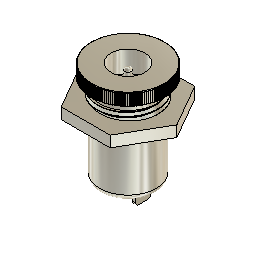
PowerConnector v3 (Autodesk Fusion 360 design; units mm, degrees)
Autodesk Fusion 360 part; units mm, degrees
sketch "Sketch1" plane through (0, 0, 0) normal (0, 0, 1) x (1, 0, 0)
  circle A0 centre (0, 0) radius 6
  circle A1 centre (0, 0) radius 2.75
  circle A2 centre (0, 0) radius 4.625
  dimension "d1" = 12
  dimension "d2" = 5.5
  dimension "d3" = 9.25
  constraint coincident A0.centre A1.centre
  constraint concentric A0 A1
  measures "d1" diameter of A0
  measures "d2" diameter of A1
  measures "d3" diameter of A2
extrude "Extrude1" add sketch "Sketch1" along normal blind 2 contours A0 | A1 | A2
extrude "Extrude2" add sketch "Sketch1" against normal blind 14.5 contours A1 | A2
fillet "Fillet1" radius 1 1 edges at (-4.312, 1.6725, -14.5)
sketch "Sketch2" plane through (0, 0, 2) normal (0, 0, 1) x (-1, 0, 0)
  circle A0 centre (0, 0) radius 6
  circle A1 centre (0, 0) radius 2.75
extrude "Extrude3" cut sketch "Sketch2" against normal blind 5 contours A1
ref_plane "WorkPlane1" through (0, 0, -3) normal (0, 0, 1) x (-1, 0, 0)
sketch "Sketch3" plane through (0, 0, -3) normal (0, 0, 1) x (1, 0, 0)
  circle A0 centre (0, 0) radius 0.5
  dimension "d15" = 1
  constraint coincident A0.centre origin
  measures "d15" diameter of A0
extrude "Extrude4" add sketch "Sketch3" along normal blind 4.5
fillet "Fillet2" radius 0.5 1 edges at (-0.4662, -0.1808, 1.5)
sketch "Sketch4" plane through (0, 0, -14.5) normal (0, 0, -1) x (1, 0, 0)
  circle A0 centre (0, 0) radius 3.625
  line L0 (-2.5, 1.25) -> (2.5, 1.25) construction
  line L1 (2.5, 1.25) -> (2.5, -1.25) construction
  line L2 (2.5, -1.25) -> (-2.5, -1.25) construction
  line L3 (-2.5, -1.25) -> (-2.5, 1.25) construction
  line L4 (-2.5, 1.25) -> (2.5, -1.25) construction
  line L5 (-2.5, 1.25) -> (-2, 1.25)
  line L6 (-2, 1.25) -> (-2, -1.25)
  line L7 (-2, -1.25) -> (-2.5, -1.25)
  line L8 (-2.5, -1.25) -> (-2.5, 1.25)
  line L9 (2.5, 1.25) -> (2, 1.25)
  line L10 (2, 1.25) -> (2, -1.25)
  line L11 (2, -1.25) -> (2.5, -1.25)
  line L12 (2.5, -1.25) -> (2.5, 1.25)
  dimension "d20" = 2.5
  dimension "d21" = 5
  dimension "d22" = 0.5
  dimension "d23" = 0.5
  constraint horizontal L0
  constraint vertical L1
  constraint horizontal L2
  constraint vertical L3
  constraint midpoint L4 A0.centre
  constraint coincident A0.centre origin
  constraint horizontal L5
  constraint vertical L6
  constraint horizontal L7
  constraint vertical L8
  constraint collinear L2 L7
  constraint horizontal L9
  constraint vertical L10
  constraint horizontal L11
  constraint vertical L12
  constraint coincident L2 L10.end
  measures "d20" distance of L0.start L2.end
  measures "d21" distance of L0.start L0.end
  measures "d22" distance of L0.start L5.end
  measures "d23" distance of L0.end L9.end
extrude "Extrude5" add sketch "Sketch4" along normal blind 2 contours L5 L6 L7 L8 | L9 L10 L11 L12
fillet "Fillet3" radius 0.5 4 edges at (-2.25, -1.25, -16.5) (-2.25, 1.25, -16.5) (2.25, -1.25, -16.5) (2.25, 1.25, -16.5)
sketch "Sketch5" plane through (0, 0, 2) normal (0, 0, 1) x (-1, 0, 0)
  circle A0 centre (0, 0) radius 2.75
  circle A1 centre (0, 0) radius 6
  circle A2 centre (0, 0) radius 6
  line L0 (0, 0) -> (-6, 0) construction
  line L1 (-5.95, -0.05) -> (-6.05, -0.05)
  line L2 (-6.05, -0.05) -> (-6.05, 0.05)
  line L3 (-6.05, 0.05) -> (-5.95, 0.05)
  line L4 (-5.95, 0.05) -> (-5.95, -0.05)
  line L5 (-5.95, -0.05) -> (-6.05, 0.05) construction
  line L6 (-5.9427, -0.2991) -> (-6.0426, -0.3033)
  line L7 (-5.9469, -0.1992) -> (-5.9427, -0.2991)
  line L8 (-6.0468, -0.2034) -> (-5.9469, -0.1992)
  line L9 (-6.0426, -0.3033) -> (-6.0468, -0.2034)
  line L10 (-5.9249, -0.5477) -> (-6.0246, -0.5561)
  line L11 (-5.9333, -0.4481) -> (-5.9249, -0.5477)
  line L12 (-6.033, -0.4564) -> (-5.9333, -0.4481)
  line L13 (-6.0246, -0.5561) -> (-6.033, -0.4564)
  line L14 (-5.8968, -0.7953) -> (-5.996, -0.8079)
  line L15 (-5.9093, -0.6961) -> (-5.8968, -0.7953)
  line L16 (-6.0086, -0.7087) -> (-5.9093, -0.6961)
  line L17 (-5.996, -0.8079) -> (-6.0086, -0.7087)
  line L18 (-5.8583, -1.0416) -> (-5.9569, -1.0583)
  line L19 (-5.875, -0.943) -> (-5.8583, -1.0416)
  line L20 (-5.9736, -0.9597) -> (-5.875, -0.943)
  line L21 (-5.9569, -1.0583) -> (-5.9736, -0.9597)
  line L22 (-5.8096, -1.286) -> (-5.9074, -1.3068)
  line L23 (-5.8304, -1.1882) -> (-5.8096, -1.286)
  line L24 (-5.9282, -1.209) -> (-5.8304, -1.1882)
  line L25 (-5.9074, -1.3068) -> (-5.9282, -1.209)
  line L26 (-5.7506, -1.5281) -> (-5.8475, -1.553)
  line L27 (-5.7755, -1.4313) -> (-5.7506, -1.5281)
  line L28 (-5.8724, -1.4561) -> (-5.7755, -1.4313)
  line L29 (-5.8475, -1.553) -> (-5.8724, -1.4561)
  line L30 (-5.6816, -1.7676) -> (-5.7773, -1.7965)
  line L31 (-5.7105, -1.6719) -> (-5.6816, -1.7676)
  line L32 (-5.8062, -1.7008) -> (-5.7105, -1.6719)
  line L33 (-5.7773, -1.7965) -> (-5.8062, -1.7008)
  line L34 (-5.6026, -2.004) -> (-5.697, -2.0369)
  line L35 (-5.6355, -1.9095) -> (-5.6026, -2.004)
  line L36 (-5.7299, -1.9424) -> (-5.6355, -1.9095)
  line L37 (-5.697, -2.0369) -> (-5.7299, -1.9424)
  line L38 (-5.5138, -2.2368) -> (-5.6067, -2.2736)
  line L39 (-5.5506, -2.1439) -> (-5.5138, -2.2368)
  line L40 (-5.6436, -2.1807) -> (-5.5506, -2.1439)
  line L41 (-5.6067, -2.2736) -> (-5.6436, -2.1807)
  line L42 (-5.4153, -2.4658) -> (-5.5066, -2.5064)
  line L43 (-5.4559, -2.3744) -> (-5.4153, -2.4658)
  line L44 (-5.5473, -2.4151) -> (-5.4559, -2.3744)
  line L45 (-5.5066, -2.5064) -> (-5.5473, -2.4151)
  line L46 (-5.3073, -2.6904) -> (-5.3968, -2.7348)
  line L47 (-5.3517, -2.6008) -> (-5.3073, -2.6904)
  line L48 (-5.4413, -2.6453) -> (-5.3517, -2.6008)
  line L49 (-5.3968, -2.7348) -> (-5.4413, -2.6453)
  line L50 (-5.1899, -2.9102) -> (-5.2776, -2.9584)
  line L51 (-5.2381, -2.8226) -> (-5.1899, -2.9102)
  line L52 (-5.3257, -2.8708) -> (-5.2381, -2.8226)
  line L53 (-5.2776, -2.9584) -> (-5.3257, -2.8708)
  line L54 (-5.0635, -3.125) -> (-5.1491, -3.1768)
  line L55 (-5.1153, -3.0395) -> (-5.0635, -3.125)
  line L56 (-5.2009, -3.0913) -> (-5.1153, -3.0395)
  line L57 (-5.1491, -3.1768) -> (-5.2009, -3.0913)
  line L58 (-4.9282, -3.3343) -> (-5.0115, -3.3897)
  line L59 (-4.9836, -3.251) -> (-4.9282, -3.3343)
  line L60 (-5.0668, -3.3064) -> (-4.9836, -3.251)
  line L61 (-5.0115, -3.3897) -> (-5.0668, -3.3064)
  line L62 (-4.7843, -3.5378) -> (-4.8652, -3.5966)
  line L63 (-4.843, -3.4569) -> (-4.7843, -3.5378)
  line L64 (-4.9239, -3.5156) -> (-4.843, -3.4569)
  line L65 (-4.8652, -3.5966) -> (-4.9239, -3.5156)
  line L66 (-4.6319, -3.735) -> (-4.7103, -3.7971)
  line L67 (-4.694, -3.6566) -> (-4.6319, -3.735)
  line L68 (-4.7724, -3.7188) -> (-4.694, -3.6566)
  line L69 (-4.7103, -3.7971) -> (-4.7724, -3.7188)
  line L70 (-4.4714, -3.9257) -> (-4.5471, -3.991)
  line L71 (-4.5368, -3.85) -> (-4.4714, -3.9257)
  line L72 (-4.6125, -3.9153) -> (-4.5368, -3.85)
  line L73 (-4.5471, -3.991) -> (-4.6125, -3.9153)
  line L74 (-4.3031, -4.1095) -> (-4.376, -4.178)
  line L75 (-4.3716, -4.0366) -> (-4.3031, -4.1095)
  line L76 (-4.4445, -4.1051) -> (-4.3716, -4.0366)
  line L77 (-4.376, -4.178) -> (-4.4445, -4.1051)
  line L78 (-4.1273, -4.2861) -> (-4.1972, -4.3575)
  line L79 (-4.1987, -4.2161) -> (-4.1273, -4.2861)
  line L80 (-4.2687, -4.2876) -> (-4.1987, -4.2161)
  line L81 (-4.1972, -4.3575) -> (-4.2687, -4.2876)
  line L82 (-3.9442, -4.4552) -> (-4.0111, -4.5295)
  line L83 (-4.0185, -4.3883) -> (-3.9442, -4.4552)
  line L84 (-4.0854, -4.4626) -> (-4.0185, -4.3883)
  line L85 (-4.0111, -4.5295) -> (-4.0854, -4.4626)
  line L86 (-3.7541, -4.6164) -> (-3.8179, -4.6935)
  line L87 (-3.8312, -4.5527) -> (-3.7541, -4.6164)
  line L88 (-3.8949, -4.6297) -> (-3.8312, -4.5527)
  line L89 (-3.8179, -4.6935) -> (-3.8949, -4.6297)
  line L90 (-3.5575, -4.7696) -> (-3.618, -4.8492)
  line L91 (-3.6372, -4.7091) -> (-3.5575, -4.7696)
  line L92 (-3.6977, -4.7888) -> (-3.6372, -4.7091)
  line L93 (-3.618, -4.8492) -> (-3.6977, -4.7888)
  line L94 (-3.3547, -4.9144) -> (-3.4118, -4.9965)
  line L95 (-3.4368, -4.8573) -> (-3.3547, -4.9144)
  line L96 (-3.4939, -4.9394) -> (-3.4368, -4.8573)
  line L97 (-3.4118, -4.9965) -> (-3.4939, -4.9394)
  line L98 (-3.146, -5.0505) -> (-3.1995, -5.135)
  line L99 (-3.2304, -4.997) -> (-3.146, -5.0505)
  line L100 (-3.284, -5.0814) -> (-3.2304, -4.997)
  line L101 (-3.1995, -5.135) -> (-3.284, -5.0814)
  line L102 (-2.9317, -5.1779) -> (-2.9817, -5.2645)
  line L103 (-3.0183, -5.1279) -> (-2.9317, -5.1779)
  line L104 (-3.0683, -5.2145) -> (-3.0183, -5.1279)
  line L105 (-2.9817, -5.2645) -> (-3.0683, -5.2145)
  line L106 (-2.7123, -5.2961) -> (-2.7586, -5.3847)
  line L107 (-2.8009, -5.2497) -> (-2.7123, -5.2961)
  line L108 (-2.8473, -5.3384) -> (-2.8009, -5.2497)
  line L109 (-2.7586, -5.3847) -> (-2.8473, -5.3384)
  line L110 (-2.4881, -5.405) -> (-2.5307, -5.4955)
  line L111 (-2.5786, -5.3624) -> (-2.4881, -5.405)
  line L112 (-2.6212, -5.4529) -> (-2.5786, -5.3624)
  line L113 (-2.5307, -5.4955) -> (-2.6212, -5.4529)
  line L114 (-2.2596, -5.5045) -> (-2.2984, -5.5966)
  line L115 (-2.3518, -5.4657) -> (-2.2596, -5.5045)
  line L116 (-2.3906, -5.5579) -> (-2.3518, -5.4657)
  line L117 (-2.2984, -5.5966) -> (-2.3906, -5.5579)
  line L118 (-2.0271, -5.5943) -> (-2.062, -5.688)
  line L119 (-2.1209, -5.5594) -> (-2.0271, -5.5943)
  line L120 (-2.1557, -5.6531) -> (-2.1209, -5.5594)
  line L121 (-2.062, -5.688) -> (-2.1557, -5.6531)
  line L122 (-1.7911, -5.6742) -> (-1.822, -5.7693)
  line L123 (-1.8862, -5.6433) -> (-1.7911, -5.6742)
  line L124 (-1.9171, -5.7384) -> (-1.8862, -5.6433)
  line L125 (-1.822, -5.7693) -> (-1.9171, -5.7384)
  line L126 (-1.5519, -5.7443) -> (-1.5788, -5.8406)
  line L127 (-1.6482, -5.7174) -> (-1.5519, -5.7443)
  line L128 (-1.6751, -5.8137) -> (-1.6482, -5.7174)
  line L129 (-1.5788, -5.8406) -> (-1.6751, -5.8137)
  line L130 (-1.31, -5.8042) -> (-1.3328, -5.9016)
  line L131 (-1.4074, -5.7814) -> (-1.31, -5.8042)
  line L132 (-1.4302, -5.8787) -> (-1.4074, -5.7814)
  line L133 (-1.3328, -5.9016) -> (-1.4302, -5.8787)
  line L134 (-1.0658, -5.854) -> (-1.0845, -5.9522)
  line L135 (-1.164, -5.8352) -> (-1.0658, -5.854)
  line L136 (-1.1828, -5.9335) -> (-1.164, -5.8352)
  line L137 (-1.0845, -5.9522) -> (-1.1828, -5.9335)
  line L138 (-0.8197, -5.8935) -> (-0.8343, -5.9924)
  line L139 (-0.9187, -5.8789) -> (-0.8197, -5.8935)
  line L140 (-0.9333, -5.9778) -> (-0.9187, -5.8789)
  line L141 (-0.8343, -5.9924) -> (-0.9333, -5.9778)
  line L142 (-0.5722, -5.9226) -> (-0.5827, -6.0221)
  line L143 (-0.6717, -5.9122) -> (-0.5722, -5.9226)
  line L144 (-0.6821, -6.0116) -> (-0.6717, -5.9122)
  line L145 (-0.5827, -6.0221) -> (-0.6821, -6.0116)
  line L146 (-0.3237, -5.9414) -> (-0.33, -6.0412)
  line L147 (-0.4235, -5.9351) -> (-0.3237, -5.9414)
  line L148 (-0.4298, -6.0349) -> (-0.4235, -5.9351)
  line L149 (-0.33, -6.0412) -> (-0.4298, -6.0349)
  line L150 (-0.0746, -5.9497) -> (-0.0767, -6.0497)
  line L151 (-0.1746, -5.9476) -> (-0.0746, -5.9497)
  line L152 (-0.1767, -6.0476) -> (-0.1746, -5.9476)
  line L153 (-0.0767, -6.0497) -> (-0.1767, -6.0476)
  line L154 (0.1746, -5.9476) -> (0.1767, -6.0476)
  line L155 (0.0746, -5.9497) -> (0.1746, -5.9476)
  line L156 (0.0767, -6.0497) -> (0.0746, -5.9497)
  line L157 (0.1767, -6.0476) -> (0.0767, -6.0497)
  line L158 (0.4235, -5.9351) -> (0.4298, -6.0349)
  line L159 (0.3237, -5.9414) -> (0.4235, -5.9351)
  line L160 (0.33, -6.0412) -> (0.3237, -5.9414)
  line L161 (0.4298, -6.0349) -> (0.33, -6.0412)
  line L162 (0.6717, -5.9122) -> (0.6821, -6.0116)
  line L163 (0.5722, -5.9226) -> (0.6717, -5.9122)
  line L164 (0.5827, -6.0221) -> (0.5722, -5.9226)
  line L165 (0.6821, -6.0116) -> (0.5827, -6.0221)
  line L166 (0.9187, -5.8789) -> (0.9333, -5.9778)
  line L167 (0.8197, -5.8935) -> (0.9187, -5.8789)
  line L168 (0.8343, -5.9924) -> (0.8197, -5.8935)
  line L169 (0.9333, -5.9778) -> (0.8343, -5.9924)
  line L170 (1.164, -5.8352) -> (1.1828, -5.9335)
  line L171 (1.0658, -5.854) -> (1.164, -5.8352)
  line L172 (1.0845, -5.9522) -> (1.0658, -5.854)
  line L173 (1.1828, -5.9335) -> (1.0845, -5.9522)
  line L174 (1.4074, -5.7814) -> (1.4302, -5.8787)
  line L175 (1.31, -5.8042) -> (1.4074, -5.7814)
  line L176 (1.3328, -5.9016) -> (1.31, -5.8042)
  line L177 (1.4302, -5.8787) -> (1.3328, -5.9016)
  line L178 (1.6482, -5.7174) -> (1.6751, -5.8137)
  line L179 (1.5519, -5.7443) -> (1.6482, -5.7174)
  line L180 (1.5788, -5.8406) -> (1.5519, -5.7443)
  line L181 (1.6751, -5.8137) -> (1.5788, -5.8406)
  line L182 (1.8862, -5.6433) -> (1.9171, -5.7384)
  line L183 (1.7911, -5.6742) -> (1.8862, -5.6433)
  line L184 (1.822, -5.7693) -> (1.7911, -5.6742)
  line L185 (1.9171, -5.7384) -> (1.822, -5.7693)
  line L186 (2.1209, -5.5594) -> (2.1557, -5.6531)
  line L187 (2.0271, -5.5943) -> (2.1209, -5.5594)
  line L188 (2.062, -5.688) -> (2.0271, -5.5943)
  line L189 (2.1557, -5.6531) -> (2.062, -5.688)
  line L190 (2.3518, -5.4657) -> (2.3906, -5.5579)
  line L191 (2.2596, -5.5045) -> (2.3518, -5.4657)
  line L192 (2.2984, -5.5966) -> (2.2596, -5.5045)
  line L193 (2.3906, -5.5579) -> (2.2984, -5.5966)
  line L194 (2.5786, -5.3624) -> (2.6212, -5.4529)
  line L195 (2.4881, -5.405) -> (2.5786, -5.3624)
  line L196 (2.5307, -5.4955) -> (2.4881, -5.405)
  line L197 (2.6212, -5.4529) -> (2.5307, -5.4955)
  line L198 (2.8009, -5.2497) -> (2.8473, -5.3384)
  line L199 (2.7123, -5.2961) -> (2.8009, -5.2497)
  line L200 (2.7586, -5.3847) -> (2.7123, -5.2961)
  line L201 (2.8473, -5.3384) -> (2.7586, -5.3847)
  line L202 (3.0183, -5.1279) -> (3.0683, -5.2145)
  line L203 (2.9317, -5.1779) -> (3.0183, -5.1279)
  line L204 (2.9817, -5.2645) -> (2.9317, -5.1779)
  line L205 (3.0683, -5.2145) -> (2.9817, -5.2645)
  line L206 (3.2304, -4.997) -> (3.284, -5.0814)
  line L207 (3.146, -5.0505) -> (3.2304, -4.997)
  line L208 (3.1995, -5.135) -> (3.146, -5.0505)
  line L209 (3.284, -5.0814) -> (3.1995, -5.135)
  line L210 (3.4368, -4.8573) -> (3.4939, -4.9394)
  line L211 (3.3547, -4.9144) -> (3.4368, -4.8573)
  line L212 (3.4118, -4.9965) -> (3.3547, -4.9144)
  line L213 (3.4939, -4.9394) -> (3.4118, -4.9965)
  line L214 (3.6372, -4.7091) -> (3.6977, -4.7888)
  line L215 (3.5575, -4.7696) -> (3.6372, -4.7091)
  line L216 (3.618, -4.8492) -> (3.5575, -4.7696)
  line L217 (3.6977, -4.7888) -> (3.618, -4.8492)
  line L218 (3.8312, -4.5527) -> (3.8949, -4.6297)
  line L219 (3.7541, -4.6164) -> (3.8312, -4.5527)
  line L220 (3.8179, -4.6935) -> (3.7541, -4.6164)
  line L221 (3.8949, -4.6297) -> (3.8179, -4.6935)
  line L222 (4.0185, -4.3883) -> (4.0854, -4.4626)
  line L223 (3.9442, -4.4552) -> (4.0185, -4.3883)
  line L224 (4.0111, -4.5295) -> (3.9442, -4.4552)
  line L225 (4.0854, -4.4626) -> (4.0111, -4.5295)
  line L226 (4.1987, -4.2161) -> (4.2687, -4.2876)
  line L227 (4.1273, -4.2861) -> (4.1987, -4.2161)
  line L228 (4.1972, -4.3575) -> (4.1273, -4.2861)
  line L229 (4.2687, -4.2876) -> (4.1972, -4.3575)
  line L230 (4.3716, -4.0366) -> (4.4445, -4.1051)
  line L231 (4.3031, -4.1095) -> (4.3716, -4.0366)
  line L232 (4.376, -4.178) -> (4.3031, -4.1095)
  line L233 (4.4445, -4.1051) -> (4.376, -4.178)
  line L234 (4.5368, -3.85) -> (4.6125, -3.9153)
  line L235 (4.4714, -3.9257) -> (4.5368, -3.85)
  line L236 (4.5471, -3.991) -> (4.4714, -3.9257)
  line L237 (4.6125, -3.9153) -> (4.5471, -3.991)
  line L238 (4.694, -3.6566) -> (4.7724, -3.7188)
  line L239 (4.6319, -3.735) -> (4.694, -3.6566)
  line L240 (4.7103, -3.7971) -> (4.6319, -3.735)
  line L241 (4.7724, -3.7188) -> (4.7103, -3.7971)
  line L242 (4.843, -3.4569) -> (4.9239, -3.5156)
  line L243 (4.7843, -3.5378) -> (4.843, -3.4569)
  line L244 (4.8652, -3.5966) -> (4.7843, -3.5378)
  line L245 (4.9239, -3.5156) -> (4.8652, -3.5966)
  line L246 (4.9836, -3.251) -> (5.0668, -3.3064)
  line L247 (4.9282, -3.3343) -> (4.9836, -3.251)
  line L248 (5.0115, -3.3897) -> (4.9282, -3.3343)
  line L249 (5.0668, -3.3064) -> (5.0115, -3.3897)
  line L250 (5.1153, -3.0395) -> (5.2009, -3.0913)
  line L251 (5.0635, -3.125) -> (5.1153, -3.0395)
  line L252 (5.1491, -3.1768) -> (5.0635, -3.125)
  line L253 (5.2009, -3.0913) -> (5.1491, -3.1768)
  line L254 (5.2381, -2.8226) -> (5.3257, -2.8708)
  line L255 (5.1899, -2.9102) -> (5.2381, -2.8226)
  line L256 (5.2776, -2.9584) -> (5.1899, -2.9102)
  line L257 (5.3257, -2.8708) -> (5.2776, -2.9584)
  line L258 (5.3517, -2.6008) -> (5.4413, -2.6453)
  line L259 (5.3073, -2.6904) -> (5.3517, -2.6008)
  line L260 (5.3968, -2.7348) -> (5.3073, -2.6904)
  line L261 (5.4413, -2.6453) -> (5.3968, -2.7348)
  line L262 (5.4559, -2.3744) -> (5.5473, -2.4151)
  line L263 (5.4153, -2.4658) -> (5.4559, -2.3744)
  line L264 (5.5066, -2.5064) -> (5.4153, -2.4658)
  line L265 (5.5473, -2.4151) -> (5.5066, -2.5064)
  line L266 (5.5506, -2.1439) -> (5.6436, -2.1807)
  line L267 (5.5138, -2.2368) -> (5.5506, -2.1439)
  line L268 (5.6067, -2.2736) -> (5.5138, -2.2368)
  line L269 (5.6436, -2.1807) -> (5.6067, -2.2736)
  line L270 (5.6355, -1.9095) -> (5.7299, -1.9424)
  line L271 (5.6026, -2.004) -> (5.6355, -1.9095)
  line L272 (5.697, -2.0369) -> (5.6026, -2.004)
  line L273 (5.7299, -1.9424) -> (5.697, -2.0369)
  line L274 (5.7105, -1.6719) -> (5.8062, -1.7008)
  line L275 (5.6816, -1.7676) -> (5.7105, -1.6719)
  line L276 (5.7773, -1.7965) -> (5.6816, -1.7676)
  line L277 (5.8062, -1.7008) -> (5.7773, -1.7965)
  line L278 (5.7755, -1.4313) -> (5.8724, -1.4561)
  line L279 (5.7506, -1.5281) -> (5.7755, -1.4313)
  line L280 (5.8475, -1.553) -> (5.7506, -1.5281)
  line L281 (5.8724, -1.4561) -> (5.8475, -1.553)
  line L282 (5.8304, -1.1882) -> (5.9282, -1.209)
  line L283 (5.8096, -1.286) -> (5.8304, -1.1882)
  line L284 (5.9074, -1.3068) -> (5.8096, -1.286)
  line L285 (5.9282, -1.209) -> (5.9074, -1.3068)
  line L286 (5.875, -0.943) -> (5.9736, -0.9597)
  line L287 (5.8583, -1.0416) -> (5.875, -0.943)
  line L288 (5.9569, -1.0583) -> (5.8583, -1.0416)
  line L289 (5.9736, -0.9597) -> (5.9569, -1.0583)
  line L290 (5.9093, -0.6961) -> (6.0086, -0.7087)
  line L291 (5.8968, -0.7953) -> (5.9093, -0.6961)
  line L292 (5.996, -0.8079) -> (5.8968, -0.7953)
  line L293 (6.0086, -0.7087) -> (5.996, -0.8079)
  line L294 (5.9333, -0.4481) -> (6.033, -0.4564)
  line L295 (5.9249, -0.5477) -> (5.9333, -0.4481)
  line L296 (6.0246, -0.5561) -> (5.9249, -0.5477)
  line L297 (6.033, -0.4564) -> (6.0246, -0.5561)
  line L298 (5.9469, -0.1992) -> (6.0468, -0.2034)
  line L299 (5.9427, -0.2991) -> (5.9469, -0.1992)
  line L300 (6.0426, -0.3033) -> (5.9427, -0.2991)
  line L301 (6.0468, -0.2034) -> (6.0426, -0.3033)
  line L302 (5.95, 0.05) -> (6.05, 0.05)
  line L303 (5.95, -0.05) -> (5.95, 0.05)
  line L304 (6.05, -0.05) -> (5.95, -0.05)
  line L305 (6.05, 0.05) -> (6.05, -0.05)
  line L306 (5.9427, 0.2991) -> (6.0426, 0.3033)
  line L307 (5.9469, 0.1992) -> (5.9427, 0.2991)
  line L308 (6.0468, 0.2034) -> (5.9469, 0.1992)
  line L309 (6.0426, 0.3033) -> (6.0468, 0.2034)
  line L310 (5.9249, 0.5477) -> (6.0246, 0.5561)
  line L311 (5.9333, 0.4481) -> (5.9249, 0.5477)
  line L312 (6.033, 0.4564) -> (5.9333, 0.4481)
  line L313 (6.0246, 0.5561) -> (6.033, 0.4564)
  line L314 (5.8968, 0.7953) -> (5.996, 0.8079)
  line L315 (5.9093, 0.6961) -> (5.8968, 0.7953)
  line L316 (6.0086, 0.7087) -> (5.9093, 0.6961)
  line L317 (5.996, 0.8079) -> (6.0086, 0.7087)
  line L318 (5.8583, 1.0416) -> (5.9569, 1.0583)
  line L319 (5.875, 0.943) -> (5.8583, 1.0416)
  line L320 (5.9736, 0.9597) -> (5.875, 0.943)
  line L321 (5.9569, 1.0583) -> (5.9736, 0.9597)
  line L322 (5.8096, 1.286) -> (5.9074, 1.3068)
  line L323 (5.8304, 1.1882) -> (5.8096, 1.286)
  line L324 (5.9282, 1.209) -> (5.8304, 1.1882)
  line L325 (5.9074, 1.3068) -> (5.9282, 1.209)
  line L326 (5.7506, 1.5281) -> (5.8475, 1.553)
  line L327 (5.7755, 1.4313) -> (5.7506, 1.5281)
  line L328 (5.8724, 1.4561) -> (5.7755, 1.4313)
  line L329 (5.8475, 1.553) -> (5.8724, 1.4561)
  line L330 (5.6816, 1.7676) -> (5.7773, 1.7965)
  line L331 (5.7105, 1.6719) -> (5.6816, 1.7676)
  line L332 (5.8062, 1.7008) -> (5.7105, 1.6719)
  line L333 (5.7773, 1.7965) -> (5.8062, 1.7008)
  line L334 (5.6026, 2.004) -> (5.697, 2.0369)
  line L335 (5.6355, 1.9095) -> (5.6026, 2.004)
  line L336 (5.7299, 1.9424) -> (5.6355, 1.9095)
  line L337 (5.697, 2.0369) -> (5.7299, 1.9424)
  line L338 (5.5138, 2.2368) -> (5.6067, 2.2736)
  line L339 (5.5506, 2.1439) -> (5.5138, 2.2368)
  line L340 (5.6436, 2.1807) -> (5.5506, 2.1439)
  line L341 (5.6067, 2.2736) -> (5.6436, 2.1807)
  line L342 (5.4153, 2.4658) -> (5.5066, 2.5064)
  line L343 (5.4559, 2.3744) -> (5.4153, 2.4658)
  line L344 (5.5473, 2.4151) -> (5.4559, 2.3744)
  line L345 (5.5066, 2.5064) -> (5.5473, 2.4151)
  line L346 (5.3073, 2.6904) -> (5.3968, 2.7348)
  line L347 (5.3517, 2.6008) -> (5.3073, 2.6904)
  line L348 (5.4413, 2.6453) -> (5.3517, 2.6008)
  line L349 (5.3968, 2.7348) -> (5.4413, 2.6453)
  line L350 (5.1899, 2.9102) -> (5.2776, 2.9584)
  line L351 (5.2381, 2.8226) -> (5.1899, 2.9102)
  line L352 (5.3257, 2.8708) -> (5.2381, 2.8226)
  line L353 (5.2776, 2.9584) -> (5.3257, 2.8708)
  line L354 (5.0635, 3.125) -> (5.1491, 3.1768)
  line L355 (5.1153, 3.0395) -> (5.0635, 3.125)
  line L356 (5.2009, 3.0913) -> (5.1153, 3.0395)
  line L357 (5.1491, 3.1768) -> (5.2009, 3.0913)
  line L358 (4.9282, 3.3343) -> (5.0115, 3.3897)
  line L359 (4.9836, 3.251) -> (4.9282, 3.3343)
  line L360 (5.0668, 3.3064) -> (4.9836, 3.251)
  line L361 (5.0115, 3.3897) -> (5.0668, 3.3064)
  line L362 (4.7843, 3.5378) -> (4.8652, 3.5966)
  line L363 (4.843, 3.4569) -> (4.7843, 3.5378)
  line L364 (4.9239, 3.5156) -> (4.843, 3.4569)
  line L365 (4.8652, 3.5966) -> (4.9239, 3.5156)
  line L366 (4.6319, 3.735) -> (4.7103, 3.7971)
  line L367 (4.694, 3.6566) -> (4.6319, 3.735)
  line L368 (4.7724, 3.7188) -> (4.694, 3.6566)
  line L369 (4.7103, 3.7971) -> (4.7724, 3.7188)
  line L370 (4.4714, 3.9257) -> (4.5471, 3.991)
  line L371 (4.5368, 3.85) -> (4.4714, 3.9257)
  line L372 (4.6125, 3.9153) -> (4.5368, 3.85)
  line L373 (4.5471, 3.991) -> (4.6125, 3.9153)
  line L374 (4.3031, 4.1095) -> (4.376, 4.178)
  line L375 (4.3716, 4.0366) -> (4.3031, 4.1095)
  line L376 (4.4445, 4.1051) -> (4.3716, 4.0366)
  line L377 (4.376, 4.178) -> (4.4445, 4.1051)
  line L378 (4.1273, 4.2861) -> (4.1972, 4.3575)
  line L379 (4.1987, 4.2161) -> (4.1273, 4.2861)
  line L380 (4.2687, 4.2876) -> (4.1987, 4.2161)
  line L381 (4.1972, 4.3575) -> (4.2687, 4.2876)
  line L382 (3.9442, 4.4552) -> (4.0111, 4.5295)
  line L383 (4.0185, 4.3883) -> (3.9442, 4.4552)
  line L384 (4.0854, 4.4626) -> (4.0185, 4.3883)
  line L385 (4.0111, 4.5295) -> (4.0854, 4.4626)
  line L386 (3.7541, 4.6164) -> (3.8179, 4.6935)
  line L387 (3.8312, 4.5527) -> (3.7541, 4.6164)
  line L388 (3.8949, 4.6297) -> (3.8312, 4.5527)
  line L389 (3.8179, 4.6935) -> (3.8949, 4.6297)
  line L390 (3.5575, 4.7696) -> (3.618, 4.8492)
  line L391 (3.6372, 4.7091) -> (3.5575, 4.7696)
  line L392 (3.6977, 4.7888) -> (3.6372, 4.7091)
  line L393 (3.618, 4.8492) -> (3.6977, 4.7888)
  line L394 (3.3547, 4.9144) -> (3.4118, 4.9965)
  line L395 (3.4368, 4.8573) -> (3.3547, 4.9144)
  line L396 (3.4939, 4.9394) -> (3.4368, 4.8573)
  line L397 (3.4118, 4.9965) -> (3.4939, 4.9394)
  line L398 (3.146, 5.0505) -> (3.1995, 5.135)
  line L399 (3.2304, 4.997) -> (3.146, 5.0505)
  line L400 (3.284, 5.0814) -> (3.2304, 4.997)
  line L401 (3.1995, 5.135) -> (3.284, 5.0814)
  line L402 (2.9317, 5.1779) -> (2.9817, 5.2645)
  line L403 (3.0183, 5.1279) -> (2.9317, 5.1779)
  line L404 (3.0683, 5.2145) -> (3.0183, 5.1279)
  line L405 (2.9817, 5.2645) -> (3.0683, 5.2145)
  line L406 (2.7123, 5.2961) -> (2.7586, 5.3847)
  line L407 (2.8009, 5.2497) -> (2.7123, 5.2961)
  line L408 (2.8473, 5.3384) -> (2.8009, 5.2497)
  line L409 (2.7586, 5.3847) -> (2.8473, 5.3384)
  line L410 (2.4881, 5.405) -> (2.5307, 5.4955)
  line L411 (2.5786, 5.3624) -> (2.4881, 5.405)
  line L412 (2.6212, 5.4529) -> (2.5786, 5.3624)
  line L413 (2.5307, 5.4955) -> (2.6212, 5.4529)
  line L414 (2.2596, 5.5045) -> (2.2984, 5.5966)
  line L415 (2.3518, 5.4657) -> (2.2596, 5.5045)
  line L416 (2.3906, 5.5579) -> (2.3518, 5.4657)
  line L417 (2.2984, 5.5966) -> (2.3906, 5.5579)
  line L418 (2.0271, 5.5943) -> (2.062, 5.688)
  line L419 (2.1209, 5.5594) -> (2.0271, 5.5943)
  line L420 (2.1557, 5.6531) -> (2.1209, 5.5594)
  line L421 (2.062, 5.688) -> (2.1557, 5.6531)
  line L422 (1.7911, 5.6742) -> (1.822, 5.7693)
  line L423 (1.8862, 5.6433) -> (1.7911, 5.6742)
  line L424 (1.9171, 5.7384) -> (1.8862, 5.6433)
  line L425 (1.822, 5.7693) -> (1.9171, 5.7384)
  line L426 (1.5519, 5.7443) -> (1.5788, 5.8406)
  line L427 (1.6482, 5.7174) -> (1.5519, 5.7443)
  line L428 (1.6751, 5.8137) -> (1.6482, 5.7174)
  line L429 (1.5788, 5.8406) -> (1.6751, 5.8137)
  line L430 (1.31, 5.8042) -> (1.3328, 5.9016)
  line L431 (1.4074, 5.7814) -> (1.31, 5.8042)
  line L432 (1.4302, 5.8787) -> (1.4074, 5.7814)
  line L433 (1.3328, 5.9016) -> (1.4302, 5.8787)
  line L434 (1.0658, 5.854) -> (1.0845, 5.9522)
  line L435 (1.164, 5.8352) -> (1.0658, 5.854)
  line L436 (1.1828, 5.9335) -> (1.164, 5.8352)
  line L437 (1.0845, 5.9522) -> (1.1828, 5.9335)
  line L438 (0.8197, 5.8935) -> (0.8343, 5.9924)
  line L439 (0.9187, 5.8789) -> (0.8197, 5.8935)
  line L440 (0.9333, 5.9778) -> (0.9187, 5.8789)
  line L441 (0.8343, 5.9924) -> (0.9333, 5.9778)
  line L442 (0.5722, 5.9226) -> (0.5827, 6.0221)
  line L443 (0.6717, 5.9122) -> (0.5722, 5.9226)
  line L444 (0.6821, 6.0116) -> (0.6717, 5.9122)
  line L445 (0.5827, 6.0221) -> (0.6821, 6.0116)
  line L446 (0.3237, 5.9414) -> (0.33, 6.0412)
  line L447 (0.4235, 5.9351) -> (0.3237, 5.9414)
  line L448 (0.4298, 6.0349) -> (0.4235, 5.9351)
  line L449 (0.33, 6.0412) -> (0.4298, 6.0349)
  line L450 (0.0746, 5.9497) -> (0.0767, 6.0497)
  line L451 (0.1746, 5.9476) -> (0.0746, 5.9497)
  line L452 (0.1767, 6.0476) -> (0.1746, 5.9476)
  line L453 (0.0767, 6.0497) -> (0.1767, 6.0476)
  line L454 (-0.1746, 5.9476) -> (-0.1767, 6.0476)
  line L455 (-0.0746, 5.9497) -> (-0.1746, 5.9476)
  line L456 (-0.0767, 6.0497) -> (-0.0746, 5.9497)
  line L457 (-0.1767, 6.0476) -> (-0.0767, 6.0497)
  line L458 (-0.4235, 5.9351) -> (-0.4298, 6.0349)
  line L459 (-0.3237, 5.9414) -> (-0.4235, 5.9351)
  line L460 (-0.33, 6.0412) -> (-0.3237, 5.9414)
  line L461 (-0.4298, 6.0349) -> (-0.33, 6.0412)
  line L462 (-0.6717, 5.9122) -> (-0.6821, 6.0116)
  line L463 (-0.5722, 5.9226) -> (-0.6717, 5.9122)
  line L464 (-0.5827, 6.0221) -> (-0.5722, 5.9226)
  line L465 (-0.6821, 6.0116) -> (-0.5827, 6.0221)
  line L466 (-0.9187, 5.8789) -> (-0.9333, 5.9778)
  line L467 (-0.8197, 5.8935) -> (-0.9187, 5.8789)
  line L468 (-0.8343, 5.9924) -> (-0.8197, 5.8935)
  line L469 (-0.9333, 5.9778) -> (-0.8343, 5.9924)
  line L470 (-1.164, 5.8352) -> (-1.1828, 5.9335)
  line L471 (-1.0658, 5.854) -> (-1.164, 5.8352)
  line L472 (-1.0845, 5.9522) -> (-1.0658, 5.854)
  line L473 (-1.1828, 5.9335) -> (-1.0845, 5.9522)
  line L474 (-1.4074, 5.7814) -> (-1.4302, 5.8787)
  line L475 (-1.31, 5.8042) -> (-1.4074, 5.7814)
  line L476 (-1.3328, 5.9016) -> (-1.31, 5.8042)
  line L477 (-1.4302, 5.8787) -> (-1.3328, 5.9016)
  line L478 (-1.6482, 5.7174) -> (-1.6751, 5.8137)
  line L479 (-1.5519, 5.7443) -> (-1.6482, 5.7174)
  line L480 (-1.5788, 5.8406) -> (-1.5519, 5.7443)
  line L481 (-1.6751, 5.8137) -> (-1.5788, 5.8406)
  line L482 (-1.8862, 5.6433) -> (-1.9171, 5.7384)
  line L483 (-1.7911, 5.6742) -> (-1.8862, 5.6433)
  line L484 (-1.822, 5.7693) -> (-1.7911, 5.6742)
  line L485 (-1.9171, 5.7384) -> (-1.822, 5.7693)
  line L486 (-2.1209, 5.5594) -> (-2.1557, 5.6531)
  line L487 (-2.0271, 5.5943) -> (-2.1209, 5.5594)
  line L488 (-2.062, 5.688) -> (-2.0271, 5.5943)
  line L489 (-2.1557, 5.6531) -> (-2.062, 5.688)
  line L490 (-2.3518, 5.4657) -> (-2.3906, 5.5579)
  line L491 (-2.2596, 5.5045) -> (-2.3518, 5.4657)
  line L492 (-2.2984, 5.5966) -> (-2.2596, 5.5045)
  line L493 (-2.3906, 5.5579) -> (-2.2984, 5.5966)
  line L494 (-2.5786, 5.3624) -> (-2.6212, 5.4529)
  line L495 (-2.4881, 5.405) -> (-2.5786, 5.3624)
  line L496 (-2.5307, 5.4955) -> (-2.4881, 5.405)
  line L497 (-2.6212, 5.4529) -> (-2.5307, 5.4955)
  line L498 (-2.8009, 5.2497) -> (-2.8473, 5.3384)
  line L499 (-2.7123, 5.2961) -> (-2.8009, 5.2497)
  line L500 (-2.7586, 5.3847) -> (-2.7123, 5.2961)
  line L501 (-2.8473, 5.3384) -> (-2.7586, 5.3847)
  line L502 (-3.0183, 5.1279) -> (-3.0683, 5.2145)
  line L503 (-2.9317, 5.1779) -> (-3.0183, 5.1279)
  line L504 (-2.9817, 5.2645) -> (-2.9317, 5.1779)
  line L505 (-3.0683, 5.2145) -> (-2.9817, 5.2645)
  line L506 (-3.2304, 4.997) -> (-3.284, 5.0814)
  line L507 (-3.146, 5.0505) -> (-3.2304, 4.997)
  line L508 (-3.1995, 5.135) -> (-3.146, 5.0505)
  line L509 (-3.284, 5.0814) -> (-3.1995, 5.135)
  line L510 (-3.4368, 4.8573) -> (-3.4939, 4.9394)
  line L511 (-3.3547, 4.9144) -> (-3.4368, 4.8573)
  line L512 (-3.4118, 4.9965) -> (-3.3547, 4.9144)
  line L513 (-3.4939, 4.9394) -> (-3.4118, 4.9965)
  line L514 (-3.6372, 4.7091) -> (-3.6977, 4.7888)
  line L515 (-3.5575, 4.7696) -> (-3.6372, 4.7091)
  line L516 (-3.618, 4.8492) -> (-3.5575, 4.7696)
  line L517 (-3.6977, 4.7888) -> (-3.618, 4.8492)
  line L518 (-3.8312, 4.5527) -> (-3.8949, 4.6297)
  line L519 (-3.7541, 4.6164) -> (-3.8312, 4.5527)
  line L520 (-3.8179, 4.6935) -> (-3.7541, 4.6164)
  line L521 (-3.8949, 4.6297) -> (-3.8179, 4.6935)
  line L522 (-4.0185, 4.3883) -> (-4.0854, 4.4626)
  line L523 (-3.9442, 4.4552) -> (-4.0185, 4.3883)
  line L524 (-4.0111, 4.5295) -> (-3.9442, 4.4552)
  line L525 (-4.0854, 4.4626) -> (-4.0111, 4.5295)
  line L526 (-4.1987, 4.2161) -> (-4.2687, 4.2876)
  line L527 (-4.1273, 4.2861) -> (-4.1987, 4.2161)
  line L528 (-4.1972, 4.3575) -> (-4.1273, 4.2861)
  line L529 (-4.2687, 4.2876) -> (-4.1972, 4.3575)
  line L530 (-4.3716, 4.0366) -> (-4.4445, 4.1051)
  line L531 (-4.3031, 4.1095) -> (-4.3716, 4.0366)
  line L532 (-4.376, 4.178) -> (-4.3031, 4.1095)
  line L533 (-4.4445, 4.1051) -> (-4.376, 4.178)
  line L534 (-4.5368, 3.85) -> (-4.6125, 3.9153)
  line L535 (-4.4714, 3.9257) -> (-4.5368, 3.85)
  line L536 (-4.5471, 3.991) -> (-4.4714, 3.9257)
  line L537 (-4.6125, 3.9153) -> (-4.5471, 3.991)
  line L538 (-4.694, 3.6566) -> (-4.7724, 3.7188)
  line L539 (-4.6319, 3.735) -> (-4.694, 3.6566)
  line L540 (-4.7103, 3.7971) -> (-4.6319, 3.735)
  line L541 (-4.7724, 3.7188) -> (-4.7103, 3.7971)
  line L542 (-4.843, 3.4569) -> (-4.9239, 3.5156)
  line L543 (-4.7843, 3.5378) -> (-4.843, 3.4569)
  line L544 (-4.8652, 3.5966) -> (-4.7843, 3.5378)
  line L545 (-4.9239, 3.5156) -> (-4.8652, 3.5966)
  line L546 (-4.9836, 3.251) -> (-5.0668, 3.3064)
  line L547 (-4.9282, 3.3343) -> (-4.9836, 3.251)
  line L548 (-5.0115, 3.3897) -> (-4.9282, 3.3343)
  line L549 (-5.0668, 3.3064) -> (-5.0115, 3.3897)
  line L550 (-5.1153, 3.0395) -> (-5.2009, 3.0913)
  line L551 (-5.0635, 3.125) -> (-5.1153, 3.0395)
  line L552 (-5.1491, 3.1768) -> (-5.0635, 3.125)
  line L553 (-5.2009, 3.0913) -> (-5.1491, 3.1768)
  line L554 (-5.2381, 2.8226) -> (-5.3257, 2.8708)
  line L555 (-5.1899, 2.9102) -> (-5.2381, 2.8226)
  line L556 (-5.2776, 2.9584) -> (-5.1899, 2.9102)
  line L557 (-5.3257, 2.8708) -> (-5.2776, 2.9584)
  line L558 (-5.3517, 2.6008) -> (-5.4413, 2.6453)
  line L559 (-5.3073, 2.6904) -> (-5.3517, 2.6008)
  line L560 (-5.3968, 2.7348) -> (-5.3073, 2.6904)
  line L561 (-5.4413, 2.6453) -> (-5.3968, 2.7348)
  line L562 (-5.4559, 2.3744) -> (-5.5473, 2.4151)
  line L563 (-5.4153, 2.4658) -> (-5.4559, 2.3744)
  line L564 (-5.5066, 2.5064) -> (-5.4153, 2.4658)
  line L565 (-5.5473, 2.4151) -> (-5.5066, 2.5064)
  line L566 (-5.5506, 2.1439) -> (-5.6436, 2.1807)
  line L567 (-5.5138, 2.2368) -> (-5.5506, 2.1439)
  line L568 (-5.6067, 2.2736) -> (-5.5138, 2.2368)
  line L569 (-5.6436, 2.1807) -> (-5.6067, 2.2736)
  line L570 (-5.6355, 1.9095) -> (-5.7299, 1.9424)
  line L571 (-5.6026, 2.004) -> (-5.6355, 1.9095)
  line L572 (-5.697, 2.0369) -> (-5.6026, 2.004)
  line L573 (-5.7299, 1.9424) -> (-5.697, 2.0369)
  line L574 (-5.7105, 1.6719) -> (-5.8062, 1.7008)
  line L575 (-5.6816, 1.7676) -> (-5.7105, 1.6719)
  line L576 (-5.7773, 1.7965) -> (-5.6816, 1.7676)
  line L577 (-5.8062, 1.7008) -> (-5.7773, 1.7965)
  line L578 (-5.7755, 1.4313) -> (-5.8724, 1.4561)
  line L579 (-5.7506, 1.5281) -> (-5.7755, 1.4313)
  line L580 (-5.8475, 1.553) -> (-5.7506, 1.5281)
  line L581 (-5.8724, 1.4561) -> (-5.8475, 1.553)
  line L582 (-5.8304, 1.1882) -> (-5.9282, 1.209)
  line L583 (-5.8096, 1.286) -> (-5.8304, 1.1882)
  line L584 (-5.9074, 1.3068) -> (-5.8096, 1.286)
  line L585 (-5.9282, 1.209) -> (-5.9074, 1.3068)
  line L586 (-5.875, 0.943) -> (-5.9736, 0.9597)
  line L587 (-5.8583, 1.0416) -> (-5.875, 0.943)
  line L588 (-5.9569, 1.0583) -> (-5.8583, 1.0416)
  line L589 (-5.9736, 0.9597) -> (-5.9569, 1.0583)
  line L590 (-5.9093, 0.6961) -> (-6.0086, 0.7087)
  line L591 (-5.8968, 0.7953) -> (-5.9093, 0.6961)
  line L592 (-5.996, 0.8079) -> (-5.8968, 0.7953)
  line L593 (-6.0086, 0.7087) -> (-5.996, 0.8079)
  line L594 (-5.9333, 0.4481) -> (-6.033, 0.4564)
  line L595 (-5.9249, 0.5477) -> (-5.9333, 0.4481)
  line L596 (-6.0246, 0.5561) -> (-5.9249, 0.5477)
  line L597 (-6.033, 0.4564) -> (-6.0246, 0.5561)
  line L598 (-5.9469, 0.1992) -> (-6.0468, 0.2034)
  line L599 (-5.9427, 0.2991) -> (-5.9469, 0.1992)
  line L600 (-6.0426, 0.3033) -> (-5.9427, 0.2991)
  line L601 (-6.0468, 0.2034) -> (-6.0426, 0.3033)
  point P0 (-6, 0)
  dimension "d28" = 0.1
  dimension "d29" = 0.1
  dimension "d31" = 360
  constraint coincident A0.centre A1.centre
  constraint coincident A2 P0
  constraint horizontal L0
  constraint horizontal L1
  constraint vertical L2
  constraint horizontal L3
  constraint vertical L4
  constraint midpoint L5 P0
  constraint coincident P0 L0.end
  measures "d28" distance of L1.start L3.end
  measures "d29" distance of L1.start L1.end
fillet "Fillet4" radius 0.1 2 edges at (-5.594, -2.1697, 2) (-5.594, -2.1697, 0)
extrude "Extrude6" cut sketch "Sketch5" against normal blind 2 contours A1 A2 L302 L303 L304 | A1 A2 L306 L307 L308 | A1 A2 L298 L299 L300 | A1 A2 L310 L311 L312 | A1 A2 L294 L295 L296 | A1 A2 L314 L315 L316 | A1 A2 L290 L291 L292 | A1 A2 L318 L319 L320 | A1 A2 L286 L287 L288 | A1 A2 L322 L323 L324 | A1 A2 L282 L283 L284 | A1 A2 L326 L327 L328 | A1 A2 L278 L279 L280 | A1 A2 L330 L331 L332 | A1 A2 L274 L275 L276 | A1 A2 L334 L335 L336 | A1 A2 L270 L271 L272 | A1 A2 L338 L339 L340 | A1 A2 L266 L267 L268 | A1 A2 L342 L343 L344 | A1 A2 L262 L263 L264 | A1 A2 L346 L347 L348 | A1 A2 L258 L259 L260 | A1 A2 L350 L351 L352 | A1 A2 L254 L255 L256 | A1 A2 L354 L355 L356 | A1 A2 L250 L251 L252 | A1 A2 L358 L359 L360 | A1 A2 L246 L247 L248 | A1 A2 L362 L363 L364 | A1 A2 L242 L243 L244 | A1 A2 L366 L367 L368 | A1 A2 L238 L239 L240 | A1 A2 L370 L371 L372 | A1 A2 L234 L235 L236 | A1 A2 L374 L375 L376 | A1 A2 L230 L231 L232 | A1 A2 L378 L379 L380 | A1 A2 L226 L227 L228 | A1 A2 L382 L383 L384 | A1 A2 L222 L223 L224 | A1 A2 L386 L387 L388 | A1 A2 L218 L219 L220 | A1 A2 L390 L391 L392 | A1 A2 L214 L215 L216 | A1 A2 L394 L395 L396 | A1 A2 L210 L211 L212 | A1 A2 L398 L399 L400 | A1 A2 L206 L207 L208 | A1 A2 L402 L403 L404 | A1 A2 L202 L203 L204 | A1 A2 L406 L407 L408 | A1 A2 L198 L199 L200 | A1 A2 L410 L411 L412 | A1 A2 L194 L195 L196 | A1 A2 L414 L415 L416 | A1 A2 L190 L191 L192 | A1 A2 L418 L419 L420 | A1 A2 L186 L187 L188 | A1 A2 L422 L423 L424 | A1 A2 L182 L183 L184 | A1 A2 L426 L427 L428 | A1 A2 L178 L179 L180 | A1 A2 L430 L431 L432 | A1 A2 L174 L175 L176 | A1 A2 L434 L435 L436 | A1 A2 L170 L171 L172 | A1 A2 L438 L439 L440 | A1 A2 L166 L167 L168 | A1 A2 L442 L443 L444 | A1 A2 L162 L163 L164 | A1 A2 L446 L447 L448 | A1 A2 L158 L159 L160 | A1 A2 L450 L451 L452 | A1 A2 L154 L155 L156 | A1 A2 L454 L455 L456 | A1 A2 L150 L151 L152 | A1 A2 L458 L459 L460 | A1 A2 L146 L147 L148 | A1 A2 L462 L463 L464 | A1 A2 L142 L143 L144 | A1 A2 L466 L467 L468 | A1 A2 L138 L139 L140 | A1 A2 L470 L471 L472 | A1 A2 L134 L135 L136 | A1 A2 L474 L475 L476 | A1 A2 L130 L131 L132 | A1 A2 L478 L479 L480 | A1 A2 L126 L127 L128 | A1 A2 L482 L483 L484 | A1 A2 L122 L123 L124 | A1 A2 L486 L487 L488 | A1 A2 L118 L119 L120 | A1 A2 L490 L491 L492 | A1 A2 L114 L115 L116 | A1 A2 L494 L495 L496 | A1 A2 L110 L111 L112 | A1 A2 L498 L499 L500 | A1 A2 L106 L107 L108 | A1 A2 L502 L503 L504 | A1 A2 L102 L103 L104 | A1 A2 L506 L507 L508 | A1 A2 L98 L99 L100 | A1 A2 L510 L511 L512 | A1 A2 L94 L95 L96 | A1 A2 L514 L515 L516 | A1 A2 L90 L91 L92 | A1 A2 L518 L519 L520 | A1 A2 L86 L87 L88 | A1 A2 L522 L523 L524 | A1 A2 L82 L83 L84 | A1 A2 L526 L527 L528 | A1 A2 L78 L79 L80 | A1 A2 L530 L531 L532 | A1 A2 L74 L75 L76 | A1 A2 L534 L535 L536 | A1 A2 L70 L71 L72 | A1 A2 L538 L539 L540 | A1 A2 L66 L67 L68 | A1 A2 L542 L543 L544 | A1 A2 L62 L63 L64 | A1 A2 L546 L547 L548 | A1 A2 L58 L59 L60 | A1 A2 L550 L551 L552 | A1 A2 L54 L55 L56 | A1 A2 L554 L555 L556 | A1 A2 L50 L51 L52 | A1 A2 L558 L559 L560 | A1 A2 L46 L47 L48 | A1 A2 L562 L563 L564 | A1 A2 L42 L43 L44 | A1 A2 L566 L567 L568 | A1 A2 L38 L39 L40 | A1 A2 L570 L571 L572 | A1 A2 L34 L35 L36 | A1 A2 L574 L575 L576 | A1 A2 L30 L31 L32 | A1 A2 L578 L579 L580 | A1 A2 L26 L27 L28 | A1 A2 L582 L583 L584 | A1 A2 L22 L23 L24 | A1 A2 L586 L587 L588 | A1 A2 L18 L19 L20 | A1 A2 L590 L591 L592 | A1 A2 L14 L15 L16 | A1 A2 L594 L595 L596 | A1 A2 L10 L11 L12 | A1 A2 L598 L599 L600 | A1 A2 L6 L7 L8 | A1 A2 L1 L3 L4
ref_plane "WorkPlane2" through (0, 0, -1.5) normal (0, 0, 1) x (1, 0, 0)
sketch "Sketch6" plane through (0, 0, -1.5) normal (0, 0, 1) x (1, 0, 0)
  circle A0 centre (0, 0) radius 5.375
  dimension "d37" = 10.75
  constraint coincident A0.centre origin
  measures "d37" diameter of A0
extrude "Extrude7" add sketch "Sketch6" against normal blind 4.5
thread "Thread2" "ISO Metric profile 10.0 M10x0.75 6g" major diameter 9.908 minor diameter 9.0475 pitch 0.75 angle 60 modelled right hand crest width 0.1054 on face at (5.3683, -0.2679, -4.5) crest through (4.954, 0, -1.3125)
ref_plane "WorkPlane3" through (0, 0, -2.8) normal (0, 0, 1) x (1, 0, 0)
sketch "Sketch7" plane through (0, 0, -2.8) normal (0, 0, 1) x (1, 0, 0)
  line L0 (0, 0) -> (8, 0) construction
  line L1 (8, 0) -> (4, 6.9282)
  line L2 (4, 6.9282) -> (-4, 6.9282)
  line L3 (-4, 6.9282) -> (-8, 0)
  line L4 (-8, 0) -> (-4, -6.9282)
  line L5 (-4, -6.9282) -> (4, -6.9282)
  line L6 (4, -6.9282) -> (8, 0)
  dimension "d41" = 8
  constraint coincident L0.start origin
  constraint horizontal L0
  constraint coincident L0.end L1.start
  measures "d41" distance of L0.start L0.end
extrude "Extrude8" add sketch "Sketch7" against normal blind 1.8
